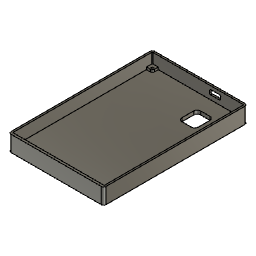
Tenkey PlusPlus Case (Autodesk Fusion 360 design; units mm, degrees)
Autodesk Fusion 360 part; units mm, degrees
note: some values were not read from the file. Set by a fixed rule: which sketch regions a step uses.
sketch "Sketch11" plane through (0, 120.2, 0) normal (0, -1, 0) x (1, 0, 0)
  line L0 (79.7, -7.05) -> (79.7, 3.5)
  line L1 (79.7, 3.5) -> (1.3, 3.5)
  line L2 (1.3, 3.5) -> (1.3, -7.05)
  line L3 (1.3, -7.05) -> (79.7, -7.05)
  line L4 (51.2, 0.6) -> (58.7, 0.6)
  line L5 (59.7, -0.4) -> (59.7, -2.3)
  line L6 (58.7, -3.3) -> (51.2, -3.3)
  line L7 (50.2, -2.3) -> (50.2, -0.4)
  line L8 (79.2, 1.5) -> (79.2, 0)
  arc A0 (51.2, 0.6) -> (50.2, -0.4) centre (51.2, -0.4) ccw
  arc A1 (59.7, -0.4) -> (58.7, 0.6) centre (58.7, -0.4) ccw
  arc A2 (58.7, -3.3) -> (59.7, -2.3) centre (58.7, -2.3) ccw
  arc A3 (50.2, -2.3) -> (51.2, -3.3) centre (51.2, -2.3) ccw
  point P0 (50.2, 0.6)
  point P1 (59.7, 0.6)
  dimension "d1" = 29
  dimension "d2" = 1
  dimension "d3" = 2.9
  dimension "d4" = 3.9
  dimension "d5" = 9.5
  constraint horizontal L4
  constraint vertical L5
  constraint horizontal L6
  constraint vertical L7
  constraint coincident P0 L4
  constraint coincident P0 L7
  constraint tangent L4 A0
  constraint tangent L7 A0
  constraint coincident P1 L5
  constraint coincident P1 L4
  constraint tangent L5 A1
  constraint tangent L4 A1
  constraint equal A0 A1
  constraint tangent L5 A2
  constraint tangent L6 A2
  constraint equal A0 A2
  constraint tangent L6 A3
  constraint tangent L7 A3
  constraint equal A0 A3
  measures "d1" distance of L7 L8
  measures "d2" radius of A0
  measures "d3" distance of L1 L4
  measures "d4" distance of L4 L6
  measures "d5" distance of L5 L7
sketch "Sketch1" plane through (0, 0, 0) normal (0, 0, 1) x (1, 0, 0)
  line L0 (-0.2, 121.7) -> (81.2, 121.7)
  line L1 (81.2, 121.7) -> (81.2, -1.4)
  line L2 (81.2, -1.4) -> (-0.2, -1.4)
  line L3 (-0.2, -1.4) -> (-0.2, 121.7)
  line L4 (79.7, 0.6) -> (1.3, 0.6)
  line L5 (1.3, 0.6) -> (1.3, 120.2)
  line L6 (1.3, 120.2) -> (79.7, 120.2)
  line L7 (79.7, 120.2) -> (79.7, 0.6)
  line L8 (3.8, 119.7) -> (77.2, 119.7)
  line L9 (1.8, 3.6) -> (1.8, 117.7)
  line L10 (79.2, 117.7) -> (79.2, 3.6)
  line L11 (77.2, 1.6) -> (3.8, 1.6)
  dimension "d43" = 0.5
  dimension "d44" = 0.5
  dimension "d45" = 0.5
  dimension "d46" = 1
  dimension "d47" = 2
  dimension "d48" = 1.5
  dimension "d49" = 1.5
  dimension "d50" = 1.5
  constraint horizontal L0
  constraint vertical L1
  constraint horizontal L2
  constraint vertical L3
  constraint horizontal L4
  constraint vertical L5
  constraint horizontal L6
  constraint vertical L7
  measures "d43" distance of L6 L8
  measures "d44" distance of L5 L9
  measures "d45" distance of L7 L10
  measures "d46" distance of L4 L11
  measures "d47" distance of L2 L4
  measures "d48" distance of L1 L7
  measures "d49" distance of L0 L6
  measures "d50" distance of L3 L5
extrude "Extrude1" add sketch "Sketch1" along normal blind 3.5 and the other way blind 7.05
sketch "Sketch2" plane through (0, 0, -7.05) normal (0, 0, -1) x (1, 0, 0)
  line L0 (79.7, -120.2) -> (1.3, -120.2)
  line L1 (1.3, -120.2) -> (1.3, -0.6)
  line L2 (1.3, -0.6) -> (79.7, -0.6)
  line L3 (79.7, -0.6) -> (79.7, -120.2)
  line L4 (81.2, 1.4) -> (-0.2, 1.4)
  line L5 (-0.2, 1.4) -> (-0.2, -121.7)
  line L6 (-0.2, -121.7) -> (81.2, -121.7)
  line L7 (81.2, -121.7) -> (81.2, 1.4)
  line L8 (81.2, -121.7) -> (-0.2, -121.7)
  line L9 (-0.2, -121.7) -> (-0.2, 1.4)
  line L10 (-0.2, 1.4) -> (81.2, 1.4)
  line L11 (81.2, 1.4) -> (81.2, -121.7)
  constraint horizontal L8
  constraint vertical L9
  constraint horizontal L10
  constraint vertical L11
  constraint coincident L4.end L5.start
  constraint coincident L6.end L7.start
extrude "Extrude2" add sketch "Sketch2" along normal blind 3 contours L0 L1 L2 L3 | L4 L5 L6 L7 L8 L9 L10 L11
sketch "Sketch3" plane through (81.2, 0, 0) normal (1, 0, 0) x (0, 1, 0)
  line L0 (121.7, -10.05) -> (121.7, 3.5)
  line L1 (121.7, 3.5) -> (-1.4, 3.5)
  line L2 (-1.4, 3.5) -> (-1.4, -10.05)
  line L3 (-1.4, -10.05) -> (121.7, -10.05)
  line L4 (121.7, -10.05) -> (121.7, -20.8199)
  line L5 (121.7, -20.8199) -> (-1.4, -10.05)
  dimension "d57" = 5
  constraint coincident L0.start L3.end
  constraint perpendicular L3 L4
  constraint coincident L2.end L3.start
  measures "d57" angle of L3 L5
extrude "Extrude3" [suppressed]
sketch "Sketch4" plane through (0, 0, -7.05) normal (0, 0, 1) x (-1, 0, 0)
  line L0 (-1.3, -120.2) -> (-1.3, -0.6)
  line L1 (-1.3, -0.6) -> (-79.7, -0.6)
  line L2 (-79.7, -0.6) -> (-79.7, -120.2)
  line L3 (-79.7, -120.2) -> (-1.3, -120.2)
  circle A0 centre (-4.7, -116.9) radius 1.75
  circle A1 centre (-4.7, -116.9) radius 1.75
  circle A2 centre (-76.3, -116.9) radius 1.75
  circle A3 centre (-4.7, -4.5) radius 1.6606
  circle A4 centre (-76.3, -116.9) radius 1.75
  circle A5 centre (-76.3, -4.5) radius 1.6606
  circle A6 centre (-4.7, -4.5) radius 1.6606
  circle A7 centre (-76.3, -4.5) radius 1.6606
  constraint coincident A0.centre A1.centre
  constraint equal A0 A1
  constraint concentric A2 A4
  constraint equal A2 A4
  constraint coincident A3.centre A6.centre
  constraint equal A3 A6
  constraint coincident A5.centre A7.centre
  constraint equal A5 A7
extrude "Extrude4" add sketch "Sketch4" along normal blind 1.95 contours A0 A1 | A2 A4 | A3 A6 | A5 A7
sketch "Sketch6" plane through (0, 0, -7.05) normal (0, 0, 1) x (-1, 0, 0)
  circle A0 centre (-4.7, -4.5) radius 1.6606
  circle A1 centre (-4.7, -116.9) radius 1.75
  circle A2 centre (-76.3, -4.5) radius 1.6606
  circle A3 centre (-76.3, -116.9) radius 1.75
  line L0 (-1.3, -120.2) -> (-1.3, -0.6)
  line L1 (-1.3, -0.6) -> (-79.7, -0.6)
  line L2 (-79.7, -0.6) -> (-79.7, -120.2)
  line L3 (-79.7, -120.2) -> (-1.3, -120.2)
  point P0 (-4.7, -116.9)
  point P1 (-76.3, -116.9)
  point P2 (-76.3, -4.5)
  point P3 (-4.7, -4.5)
  constraint coincident P0 A1.centre
  constraint coincident P1 A3.centre
  constraint coincident P2 A2.centre
  constraint coincident P3 A0.centre
hole "Hole2" at (76.3, 116.9, -5.1) direction (0, 0, -1) diameter 1.9 depth 3.5 tip angle 118
hole "Hole3" at (4.7, 116.9, -5.1) direction (0, 0, -1) diameter 1.9 depth 3.5 tip angle 118
hole "Hole4" at (4.7, 4.5, -5.1) direction (0, 0, -1) diameter 1.9 depth 3.5 tip angle 118
hole "Hole5" at (76.3, 4.5, -5.1) direction (0, 0, -1) diameter 1.9 depth 3.5 tip angle 118
fillet "Fillet1" [suppressed]
extrude "Extrude5" cut sketch "Sketch11" against normal through all contours L4 L5 L6 L7 A0 A1 A2 A3
fillet "Fillet2" radius 2 4 edges at (81.2, -1.4, -3.275) (-0.2, -1.4, -3.275) (81.2, 121.7, -3.275) (-0.2, 121.7, -3.275)
fillet "Fillet3" radius 0.5 4 edges at (1.3, 120.2, -1.775) (79.7, 120.2, -1.775) (1.3, 0.6, -1.775) (79.7, 0.6, -1.775)
sketch "Sketch7" plane through (0, 0, -7.05) normal (0, 0, 1) x (-1, 0, 0)
  arc A0 (-79.2, -0.6) -> (-79.7, -1.1) centre (-79.2, -1.1) ccw
  line L0 (-79.7, -1.1) -> (-79.7, -119.7)
  arc A1 (-79.7, -119.7) -> (-79.2, -120.2) centre (-79.2, -119.7) ccw
  line L1 (-79.2, -120.2) -> (-1.8, -120.2)
  arc A2 (-1.8, -120.2) -> (-1.3, -119.7) centre (-1.8, -119.7) ccw
  line L2 (-1.3, -119.7) -> (-1.3, -1.1)
  arc A3 (-1.3, -1.1) -> (-1.8, -0.6) centre (-1.8, -1.1) ccw
  line L3 (-1.8, -0.6) -> (-79.2, -0.6)
  circle A4 centre (-76.3, -116.9) radius 1.75
  circle A5 centre (-76.3, -4.5) radius 1.6606
  circle A6 centre (-4.7, -116.9) radius 1.75
  circle A7 centre (-4.7, -4.5) radius 1.6606
  line L4 (-55.2, -107.7) -> (-63.2, -107.7)
  line L5 (-66.2, -104.7) -> (-66.2, -94.7)
  line L6 (-63.2, -91.7) -> (-55.2, -91.7)
  line L7 (-52.2, -94.7) -> (-52.2, -104.7)
  line L8 (-3.8, -119.7) -> (-77.2, -119.7)
  line L9 (-1.8, -3.6) -> (-1.8, -117.7)
  arc A8 (-55.2, -107.7) -> (-52.2, -104.7) centre (-55.2, -104.7) ccw
  arc A9 (-66.2, -104.7) -> (-63.2, -107.7) centre (-63.2, -104.7) ccw
  arc A10 (-63.2, -91.7) -> (-66.2, -94.7) centre (-63.2, -94.7) ccw
  arc A11 (-52.2, -94.7) -> (-55.2, -91.7) centre (-55.2, -94.7) ccw
  line L10 (-79.2, -117.7) -> (-79.2, -3.6)
  line L11 (-55.2, -104.7) -> (-63.2, -94.7) construction
  line L12 (-55.2, -94.7) -> (-63.2, -104.7) construction
  point P0 (-59.2, -99.7)
  dimension "d91" = 12
  dimension "d95" = 3
  dimension "d98" = 14
  dimension "d104" = 20
  dimension "d105" = 20
  constraint horizontal L4
  constraint vertical L5
  constraint horizontal L6
  constraint vertical L7
  constraint tangent L4 A8
  constraint tangent L7 A8
  constraint tangent L4 A9
  constraint tangent L5 A9
  constraint equal A8 A9
  constraint tangent L5 A10
  constraint tangent L6 A10
  constraint equal A8 A10
  constraint tangent L6 A11
  constraint tangent L7 A11
  constraint equal A8 A11
  constraint coincident A8.centre L11.start
  constraint coincident A10.centre L11.end
  constraint coincident A11.centre L12.start
  constraint coincident A9.centre L12.end
  constraint midpoint L12 P0
  measures "d91" distance of L4 L8
  measures "d95" radius of A8
  measures "d98" distance of L5 L7
  measures "d104" distance of L10 P0
  measures "d105" distance of L8 P0
extrude "Extrude6" cut sketch "Sketch7" against normal through all contours L4 L5 L6 L7 A8 A9 A10 A11
sketch "Sketch10" plane through (0, 0, -7.05) normal (0, 0, 1) x (-1, 0, 0)
  line L0 (-66.2, -104.7) -> (-66.2, -94.7)
  arc A0 (-63.2, -91.7) -> (-66.2, -94.7) centre (-63.2, -94.7) ccw
  line L1 (-63.2, -91.7) -> (-55.2, -91.7)
  arc A1 (-52.2, -94.7) -> (-55.2, -91.7) centre (-55.2, -94.7) ccw
  line L2 (-52.2, -94.7) -> (-52.2, -104.7)
  arc A2 (-55.2, -107.7) -> (-52.2, -104.7) centre (-55.2, -104.7) ccw
  line L3 (-55.2, -107.7) -> (-63.2, -107.7)
  arc A3 (-66.2, -104.7) -> (-63.2, -107.7) centre (-63.2, -104.7) ccw
  arc A4 (-79.2, -0.6) -> (-79.7, -1.1) centre (-79.2, -1.1) ccw
  line L4 (-79.7, -1.1) -> (-79.7, -119.7)
  arc A5 (-79.7, -119.7) -> (-79.2, -120.2) centre (-79.2, -119.7) ccw
  line L5 (-79.2, -120.2) -> (-1.8, -120.2)
  arc A6 (-1.8, -120.2) -> (-1.3, -119.7) centre (-1.8, -119.7) ccw
  line L6 (-1.3, -119.7) -> (-1.3, -1.1)
  arc A7 (-1.3, -1.1) -> (-1.8, -0.6) centre (-1.8, -1.1) ccw
  line L7 (-1.8, -0.6) -> (-79.2, -0.6)
  circle A8 centre (-76.3, -116.9) radius 1.75
  circle A9 centre (-76.3, -4.5) radius 1.6606
  circle A10 centre (-4.7, -116.9) radius 1.75
  circle A11 centre (-4.7, -4.5) radius 1.6606
  line L8 (-6.3606, -4.5) -> (-6.3606, -0.6)
  line L9 (-4.7, -6.1606) -> (-1.3, -6.1606)
  arc A12 (-4.7, -6.1606) -> (-6.3606, -4.5) centre (-4.7, -4.5) ccw
  circle A13 centre (-4.7, -4.5) radius 0.95
  line L10 (-74.6394, -4.5) -> (-74.6394, -0.6)
  line L11 (-76.3, -6.1606) -> (-79.7, -6.1606)
  line L12 (-76.3, -115.15) -> (-79.7, -115.15)
  line L13 (-74.55, -116.9) -> (-74.55, -120.2)
  line L14 (-6.45, -116.9) -> (-6.45, -120.2)
  line L15 (-4.7, -115.15) -> (-1.3, -115.15)
  constraint coincident A11 L8.start
  constraint coincident L7 L8.end
  constraint tangent A11 L8
  constraint coincident A11 L9.start
  constraint coincident L6 L9.end
  constraint perpendicular L6 L9
  constraint tangent A11 L9
  constraint concentric A12 A13
  constraint perpendicular L7 L8
  constraint coincident A9 L10.start
  constraint coincident L7 L10.end
  constraint coincident A9 L11.start
  constraint coincident L4 L11.end
  constraint perpendicular L4 L11
  constraint tangent A9 L11
  constraint tangent A9 L10
  constraint perpendicular L7 L10
  constraint coincident A8 L12.start
  constraint coincident L4 L12.end
  constraint tangent A8 L12
  constraint coincident A8 L13.start
  constraint coincident L5 L13.end
  constraint tangent A8 L13
  constraint perpendicular L5 L13
  constraint perpendicular L4 L12
  constraint coincident A10 L14.start
  constraint coincident L5 L14.end
  constraint tangent A10 L14
  constraint coincident A10 L15.start
  constraint coincident L6 L15.end
  constraint tangent A10 L15
  constraint perpendicular L6 L15
  constraint perpendicular L5 L14
extrude "Extrude7" add sketch "Sketch10" along normal blind 1.95 contours A4 L4 L7 A9 L10 L11 | L6 A7 L7 A11 L8 L9 A12 | L4 A5 L5 A8 L12 L13 | L5 A6 L6 A10 L14 L15
equation "d53 = 3.5 mm + 3.55 mm"
equation "d60 = 3.55 mm - 1.6 mm"
